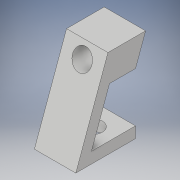
# Autodesk Inventor part: camera-brackets-angle
Saved by Autodesk Inventor 2019 (Build 230136000, 136)
## iProperties
Created: 2019-04-19
Part Number: camera-brackets-angle
Material: Generic
Document SubType Name: Modeling
Designer: Tesler
Density: 1 g/cm^3
Appearance: Default
Author: Tesler
## iProperties of the stored document camera-brackets-angle_3DPrint.ipt
Created: 2019-04-22
Part Number: camera-brackets-angle_3DPrint
Material: Generic
Document SubType Name: Modeling
Designer: Tesler
Density: 1 g/cm^3
Appearance: Default
Author: Tesler
Autodesk Inventor part; units mm, degrees
ref_plane "YZ Plane" through (0, 0, 0) normal (1, 0, 0) x (0, 1, 0)
ref_plane "XZ Plane" through (0, 0, 0) normal (0, 1, 0) x (-1, 0, 0)
ref_plane "XY Plane" through (0, 0, 0) normal (0, 0, 1) x (1, 0, 0)
sketch "Sketch1" plane through (0, 0, 0) normal (1, 0, 0) x (0, 1, 0)
  line L0 (0, 0) -> (15, -5.4596)
  line L1 (0, 0) -> (0, -9.4596)
  line L2 (15, -5.4596) -> (15, -9.4596)
  line L3 (15, -9.4596) -> (0, -9.4596)
  dimension "d12" = 70
  dimension "d17" = 15
  dimension "d18" = 4
  constraints: 8 end point, 3 vertical, 1 horizontal, 1 perpendicular
  measures "d12" angle of L1 L0
  measures "d17" horizontal distance of L0.start L0.end
  measures "d18" distance of L0.end L2.end
extrude "Extrusion1" add sketch "Sketch1" along normal blind 7.5
sketch "Sketch2" plane through (7.5, 0, 0) normal (1, 0, 0) x (0, 0, -1)
  line L0 (9.4596, 0) -> (9.4596, 15) projected
  line L1 (9.4596, 1) -> (1.4596, 1)
  line L2 (0, 0) -> (9.4596, 0) projected
  line L3 (1.4596, 1) -> (4.7353, 10)
  line L4 (9.4596, 10) -> (4.7353, 10)
  line L5 (9.4596, 1) -> (9.4596, 10)
  point P0 (5.4596, 15)
  dimension "d23" = 8
  dimension "d24" = 10
  dimension "d25" = 70
  dimension "d26" = 4.7243
  constraints: 8 end point, 2 horizontal, 2 point on line, 1 collinear
  measures "d23" distance of L1.start L1.end
  measures "d24" distance between parallel lines of L4 L2
  measures "d25" angle of L1 L3
  measures "d26" distance of L4.start L3.end
extrude "Extrusion2" cut sketch "Sketch2" against normal blind 10
sketch "Sketch5" plane through (0, 0, 0) normal (-1, 0, 0) x (0, 0, 1)
  line L0 (-5.4596, 15) -> (-9.4596, 15) projected
  line L1 (-9.4596, 10) -> (-4.7353, 10) projected
  line L2 (-4.7353, 10) -> (-1.4596, 1) projected
  line L3 (-1.4596, 1) -> (-9.4596, 1) projected
  line L4 (-9.4596, 1) -> (-9.4596, 0) projected
  line L5 (-9.4596, 0) -> (0, 0) projected
  line L6 (0, 0) -> (-5.4596, 15) projected
  line L7 (-5.4596, 15) -> (-9.4596, 15) projected
  line L8 (-9.4596, 15) -> (-9.4596, 10) projected
  line L9 (-9.4596, 10) -> (-11.2794, 15)
  line L10 (-5.4596, 15) -> (0, 0) projected
  line L11 (-9.4596, 10) -> (-9.4596, 15) projected
  line L12 (-9.4596, 10) -> (-9.4596, 15)
  line L13 (-9.4596, 15) -> (-11.2794, 15)
  constraints: 6 end point, 1 collinear, 1 horizontal, 1 parallel
extrude "Extrusion5" add sketch "Sketch5" against normal up to surface (7.5 mm away) contours L8 L9 L13
sketch "Sketch6" plane through (7.5, 0, 0) normal (1, 0, 0) x (0, 0, -1)
  line L0 (5.4596, 15) -> (0, 0) projected
  line L1 (0, 0) -> (-0.364, -1)
  line L2 (9.4596, 0) -> (9.4596, 1) projected
  line L3 (9.4596, 0) -> (9.4596, -1)
  line L4 (0, 0) -> (9.4596, 0) projected
  line L5 (0, 0) -> (9.4596, 0)
  line L6 (9.4596, -1) -> (-0.364, -1)
  dimension "d41" = 1
  dimension "d42" = 70
  constraints: 8 end point, 1 collinear, 1 horizontal, 1 vertical
  measures "d41" distance of L2.start L3.end
  measures "d42" angle of L6 L1
extrude "Extrusion6" add sketch "Sketch6" against normal up to surface (7.5 mm away)
sketch "Sketch4" plane through (7.5, 1, -1.4596) normal (0, 1, 0) x (1, 0, 0)
  line L0 (-7.5, 0) -> (-7.5, 8) projected
  line L1 (-7.5, 8) -> (0, 8) projected
  circle A0 centre (-3.75, 4) radius 1.75
  point P0 (-7.5, -1.4596)
  point P1 (-7.5, 4)
  point P2 (-3.75, 8)
  dimension "d32" = 3.5
  constraints: 2 midpoint, 1 centre point, 1 horizontal alignment, 1 vertical alignment
  measures "d32" diameter of A0
extrude "Extrusion4" cut sketch "Sketch4" against normal blind 10
sketch "Sketch7" plane through (7.5, 0, 0) normal (1, 0, 0) x (0, 0, -1)
  line L0 (5.4596, 15) -> (11.2794, 15) projected
  line L1 (-0.364, -1) -> (9.4596, -1) projected
  line L2 (5.4596, 15) -> (4.4596, 15)
  line L3 (-0.364, -1) -> (-1.364, -1)
  line L4 (-1.364, -1) -> (4.4596, 15)
  line L5 (5.4596, 15) -> (-0.364, -1) projected
  line L6 (5.4596, 15) -> (-0.364, -1)
  point P0 (0, 0)
  dimension "d45" = 1
  dimension "d46" = 1
  constraints: 8 end point, 2 horizontal, 1 collinear
  measures "d45" distance of L0.start L2.end
  measures "d46" distance of L1.start L3.end
extrude "Extrusion7" add sketch "Sketch7" against normal up to surface (7.5 mm away)
sketch "Sketch3" plane through (7.5, 15, -9.4596) normal (0, 0, -1) x (-1, 0, 0)
  circle A0 centre (3.75, -2.5) radius 1.75
  line L0 (7.5, 0) -> (0, 0) projected
  line L1 (7.5, 0) -> (7.5, -5) projected
  point P0 (7.5, -15)
  point P1 (3.75, 0)
  point P2 (7.5, -2.5)
  dimension "d29" = 3.5
  constraints: 2 midpoint, 1 centre point, 1 horizontal alignment, 1 vertical alignment
  measures "d29" diameter of A0
extrude "Extrusion3" cut sketch "Sketch3" against normal blind 10 and the other way blind 5
body "Solid1"
